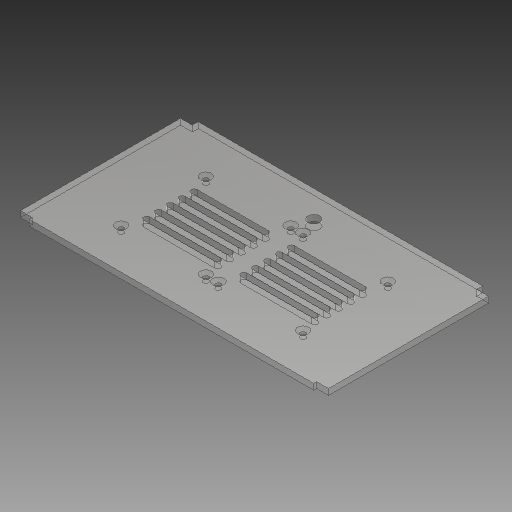
# Autodesk Inventor part: SeitenOben
Saved by Autodesk Inventor 2019 (Build 230136000, 136)
## iProperties
Created: 2018-04-27
Part Number: SeitenOben
Material: Polycarbonate, Clear
Document SubType Name: Modeling
Designer: Phil Erle
Density: 1.2 g/cm^3
Appearance: Polycarbonate - Clear
Author: Phil Erle
Autodesk Inventor part; units mm, degrees
ref_plane "YZ Plane" through (0, 0, 0) normal (1, 0, 0) x (0, 1, 0)
ref_plane "XZ Plane" through (0, 0, 0) normal (0, 1, 0) x (-1, 0, 0)
ref_plane "XY Plane" through (0, 0, 0) normal (0, 0, 1) x (1, 0, 0)
sketch "Sketch1" plane through (0, 0, 0) normal (0, 0, 1) x (1, 0, 0)
  line L0 (-130, 67.5) -> (-130, -67.5)
  line L1 (-130, -67.5) -> (-120, -67.5)
  line L2 (-120, -67.5) -> (-120, -70)
  line L3 (-120, -70) -> (120, -70)
  line L4 (120, -70) -> (120, -67.5)
  line L5 (120, -67.5) -> (130, -67.5)
  line L6 (130, -67.5) -> (130, 67.5)
  line L7 (130, 67.5) -> (120, 67.5)
  line L8 (120, 67.5) -> (120, 72.5)
  line L9 (120, 72.5) -> (-120, 72.5)
  line L10 (-120, 72.5) -> (-120, 67.5)
  line L11 (-130, 67.5) -> (-120, 67.5)
  point P0 (0, 0)
  point P1 (0, 72.5)
  point P2 (130, 0)
  point P3 (-130, 0)
  dimension "d0" = 5
  dimension "d1" = 240
  dimension "d2" = 10
  dimension "d3" = 10
  dimension "d4" = 2.5
  dimension "d5" = 135
  constraints: 24 end point, 8 perpendicular, 7 point on line, 3 midpoint, 1 horizontal alignment, 1 vertical, 1 vertical alignment
  measures "d0" distance of L7.end L8.end
  measures "d1" distance of L8.end L9.end
  measures "d2" distance of L0.start L10.end
  measures "d3" distance of L6.end L7.end
  measures "d4" distance of L3.end L4.end
  measures "d5" distance between parallel lines of L1 L11
extrude "Extrusion1" add sketch "Sketch1" along normal blind 5
sketch "Sketch2" plane through (0, 0, 5) normal (0, 0, 1) x (1, 0, 0)
  line L0 (-76.75, -35.75) -> (-5.25, -35.75) construction
  line L1 (-5.25, -35.75) -> (-5.25, 35.75) construction
  line L2 (-5.25, 35.75) -> (-76.75, 35.75) construction
  line L3 (-76.75, 35.75) -> (-76.75, -35.75) construction
  line L4 (-76.75, -35.75) -> (-5.25, 35.75) construction
  line L5 (-5.25, -35.75) -> (-76.75, 35.75) construction
  line L6 (5.25, -35.75) -> (76.75, -35.75) construction
  line L7 (76.75, -35.75) -> (76.75, 35.75) construction
  line L8 (76.75, 35.75) -> (5.25, 35.75) construction
  line L9 (5.25, 35.75) -> (5.25, -35.75) construction
  line L10 (5.25, -35.75) -> (76.75, 35.75) construction
  line L11 (76.75, -35.75) -> (5.25, 35.75) construction
  point P0 (0, 0)
  point P1 (-41, 0)
  point P2 (41, 0)
  point P3 (-41, 0)
  point P4 (41, 0)
  point P5 (76.75, 35.75)
  dimension "d8" = 71.5
  dimension "d9" = 71.5
  dimension "d10" = 71.5
  dimension "d11" = 82
  dimension "d12" = 41
  constraints: 24 end point, 8 coincident, 6 midpoint, 4 parallel, 2 horizontal, 2 horizontal alignment, 2 perpendicular, 1 point on line
  measures "d8" distance of L2.end L0.start
  measures "d9" distance of L1.end L2.end
  measures "d10" distance of L7.end L8.end
  measures "d11" distance of point (41, 0) point (-41, 0)
  measures "d12" distance of point (0, 0) point (-41, 0)
hole "Hole1" at (-76.75, 35.75, 5) at (-5.25, 35.75, 5) at (-5.25, -35.75, 5) at (-76.75, -35.75, 5) at (5.25, 35.75, 5) at (76.75, 35.75, 5) at (76.75, -35.75, 5) at (5.25, -35.75, 5) direction (0, 0, -1) diameter 4.5 depth 8 tip angle 118 countersink diameter 9.4 countersink angle 90 clearance for "Countersunk Flat Head Screw DIN EN ISO 2009" size "M4" standard "DIN"
sketch "Sketch4" plane through (0, 0, 5) normal (0, 0, 1) x (1, 0, 0)
  circle A0 centre (-76.75, 35.75) radius 2.25 projected
  circle A1 centre (-5.25, 35.75) radius 2.25 projected
  circle A2 centre (5.25, 35.75) radius 2.25 projected
  circle A3 centre (76.75, 35.75) radius 2.25 projected
  circle A4 centre (76.75, -35.75) radius 2.25 projected
  circle A5 centre (5.25, -35.75) radius 2.25 projected
  circle A6 centre (-5.25, -35.75) radius 2.25 projected
  circle A7 centre (-76.75, -35.75) radius 2.25 projected
  circle A8 centre (-5.25, -35.75) radius 2.25 construction
  line L0 (-76.75, 35.75) -> (-5.25, 35.75) construction
  line L1 (-5.25, 35.75) -> (-5.25, -35.75) construction
  line L2 (-5.25, -35.75) -> (-76.75, -35.75) construction
  line L3 (-76.75, -35.75) -> (-76.75, 35.75) construction
  line L4 (5.25, -35.75) -> (76.75, -35.75) construction
  line L5 (76.75, -35.75) -> (76.75, 35.75) construction
  line L6 (76.75, 35.75) -> (5.25, 35.75) construction
  line L7 (5.25, 35.75) -> (5.25, -35.75) construction
  line L8 (-71, 0) -> (-11, 0)
  line L9 (-71, -2.5) -> (-11, -2.5)
  line L10 (-11, 2.5) -> (-71, 2.5)
  arc A9 (-71, 2.5) -> (-71, -2.5) centre (-71, 0) ccw
  arc A10 (-11, -2.5) -> (-11, 2.5) centre (-11, 0) ccw
  line L11 (-130, 67.5) -> (-130, -67.5) construction
  arc A11 (-11, -12.5) -> (-11, -7.5) centre (-11, -10) ccw
  line L12 (-71, -10) -> (-11, -10)
  line L13 (-71, -12.5) -> (-11, -12.5)
  line L14 (-11, -7.5) -> (-71, -7.5)
  arc A12 (-71, -7.5) -> (-71, -12.5) centre (-71, -10) ccw
  arc A13 (-11, -22.5) -> (-11, -17.5) centre (-11, -20) ccw
  line L15 (-71, -20) -> (-11, -20)
  line L16 (-71, -22.5) -> (-11, -22.5)
  line L17 (-11, -17.5) -> (-71, -17.5)
  arc A14 (-71, -17.5) -> (-71, -22.5) centre (-71, -20) ccw
  line L18 (-71, 7.5) -> (-11, 7.5)
  line L19 (-71, 10) -> (-11, 10)
  line L20 (-11, 12.5) -> (-71, 12.5)
  arc A15 (-11, 7.5) -> (-11, 12.5) centre (-11, 10) ccw
  arc A16 (-71, 12.5) -> (-71, 7.5) centre (-71, 10) ccw
  line L21 (-71, 17.5) -> (-11, 17.5)
  line L22 (-71, 20) -> (-11, 20)
  line L23 (-11, 22.5) -> (-71, 22.5)
  arc A17 (-11, 17.5) -> (-11, 22.5) centre (-11, 20) ccw
  arc A18 (-71, 22.5) -> (-71, 17.5) centre (-71, 20) ccw
  line L24 (0, 82.6384) -> (0, -86.5576) construction
  line L25 (71, 0) -> (11, 0)
  line L26 (71, -2.5) -> (11, -2.5)
  line L27 (11, 2.5) -> (71, 2.5)
  arc A19 (71, -2.5) -> (71, 2.5) centre (71, 0) ccw
  arc A20 (11, 2.5) -> (11, -2.5) centre (11, 0) ccw
  arc A21 (11, -7.5) -> (11, -12.5) centre (11, -10) ccw
  line L28 (71, -10) -> (11, -10)
  line L29 (71, -12.5) -> (11, -12.5)
  line L30 (11, -7.5) -> (71, -7.5)
  arc A22 (71, -12.5) -> (71, -7.5) centre (71, -10) ccw
  arc A23 (11, -17.5) -> (11, -22.5) centre (11, -20) ccw
  line L31 (71, -20) -> (11, -20)
  line L32 (71, -22.5) -> (11, -22.5)
  line L33 (11, -17.5) -> (71, -17.5)
  arc A24 (71, -22.5) -> (71, -17.5) centre (71, -20) ccw
  line L34 (71, 7.5) -> (11, 7.5)
  line L35 (71, 10) -> (11, 10)
  line L36 (11, 12.5) -> (71, 12.5)
  arc A25 (11, 12.5) -> (11, 7.5) centre (11, 10) ccw
  arc A26 (71, 7.5) -> (71, 12.5) centre (71, 10) ccw
  line L37 (71, 17.5) -> (11, 17.5)
  line L38 (71, 20) -> (11, 20)
  line L39 (11, 22.5) -> (71, 22.5)
  arc A27 (11, 22.5) -> (11, 17.5) centre (11, 20) ccw
  arc A28 (71, 17.5) -> (71, 22.5) centre (71, 20) ccw
  point P0 (0, 0)
  point P1 (-41, 0)
  point P2 (-41, -10)
  point P3 (-41, -20)
  point P4 (-41, 10)
  point P5 (-41, 20)
  point P6 (41, 0)
  point P7 (41, -10)
  point P8 (41, -20)
  point P9 (41, 10)
  point P10 (41, 20)
  dimension "d21" = 30
  dimension "d22" = 5
  dimension "d23" = 35.75
  dimension "d26" = 10
  dimension "d33" = 10
  dimension "d38" = 35.75
  constraints: 98 end point, 40 point on circle, 35 symmetric about line, 20 centre point, 5 parallel, 4 tangent, 3 horizontal, 3 vertical, 2 perpendicular, 1 horizontal alignment, 1 midpoint, 58 other
  measures "d21" distance of point (-41, 0) L8.end
  measures "d22" diameter of A10
  measures "d23" distance from line of L1 point (-41, 0)
  measures "d26" distance of L9.end L13.end
  measures "d33" distance of L9.start L18.start
  measures "d38" distance from line of L7 point (41, 0)
extrude "Extrusion2" cut sketch "Sketch4" against normal blind 5 contours A9 L10 A10 L9 | L13 A12 L14 A11 | L16 A14 L17 A13 | A16 L20 A15 L18 | A18 L23 A17 L21 | L26 A20 L27 A19 | L30 A22 L29 A21 | L33 A24 L32 A23 | L34 A25 L36 A26 | L37 A27 L39 A28
sketch "Sketch5" plane through (0, 0, 5) normal (0, 0, 1) x (1, 0, 0)
  point P0 (0, 0)
  point P1 (0, 50)
  point P2 (0, 50)
  dimension "d42" = 50
  constraints: 1 coincident, 1 vertical alignment
  measures "d42" distance of point (0, 0) point (0, 50)
hole "Hole2" at (0, 50, 5) direction (0, 0, -1) diameter 10 depth 8 tip angle 118
equation "\"d12\" = 0.5 * d11"
equation "\"d39\" = d22"
body "Solid1"
